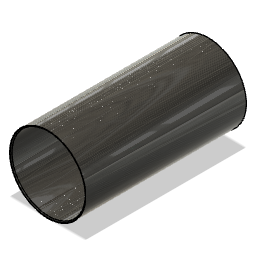
Antriebssektion 2 350 v3 (Autodesk Fusion 360 design; units mm, degrees)
Autodesk Fusion 360 part; units mm, degrees
sketch "Skizze1" plane through (0, 0, 0) normal (0, 0, 1) x (1, 0, 0)
  circle A0 centre (0, 0) radius 83
  circle A1 centre (0, 0) radius 80
  dimension "d1" = 160
  dimension "d2" = 166
  constraint coincident A0.centre A1.centre
  measures "d1" diameter of A1
  measures "d2" diameter of A0
extrude "Extrusion1" add sketch "Skizze1" along normal blind 350
fillet "Abrundung1" radius 2 2 edges at (-74.5862, 28.9292, 350) (-74.5862, 28.9292, 0)
